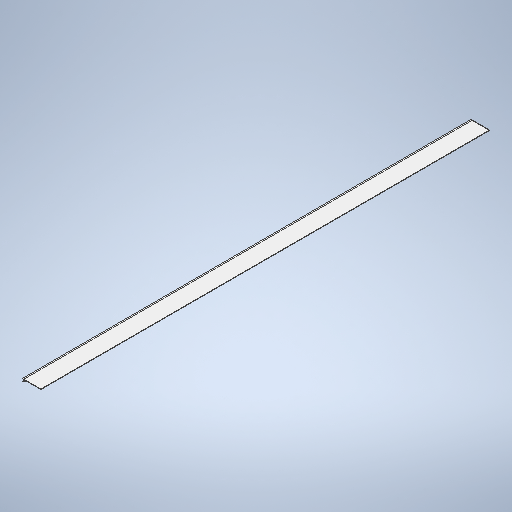
# Autodesk Inventor part: Drip_Edge_For_Side
Saved by Autodesk Inventor 2025 (Build 290162010, 162A)
## iProperties
Created: 2024-09-15
Part Number: Drip_Edge_For_Side
Material: Aluminum 6061
Document SubType Name: Modeling
Designer: Tom
Density: 2.7 g/cm^3
Appearance: White
Author: Tom
Autodesk Inventor part; units mm, degrees
ref_plane "YZ Plane" through (0, 0, 0) normal (1, 0, 0) x (0, 1, 0)
ref_plane "XZ Plane" through (0, 0, 0) normal (0, 1, 0) x (-1, 0, 0)
ref_plane "XY Plane" through (0, 0, 0) normal (0, 0, 1) x (1, 0, 0)
sketch "Sketch1" plane through (0, 0, 0) normal (0, 0, 1) x (1, 0, 0)
  line L0 (152.4, -3.175) -> (152.4, 0)
  line L1 (152.4, 0) -> (0, 0)
  line L2 (0, 0) -> (9.525, -8.4582)
  line L3 (9.525, -8.4582) -> (9.525, -16.9164)
  line L4 (9.525, -16.9164) -> (0, -22.655)
  line L5 (1.6385, -25.3746) -> (12.7, -18.7102)
  line L6 (12.7, -18.7102) -> (12.7, -7.0315)
  line L7 (12.7, -7.0315) -> (8.3571, -3.175)
  line L8 (8.3571, -3.175) -> (152.4, -3.175)
  line L9 (1.6385, -25.3746) -> (0, -22.655)
  line L10 (0, 0) -> (0, -22.655)
  dimension "d49" = 3.175
  dimension "d50" = 3.175
  dimension "d51" = 3.175
  dimension "d52" = 3.175
  dimension "d54" = 8.4582
  dimension "d55" = 8.4582
  dimension "d61" = 8.4582
  dimension "d62" = 152.4
  dimension "d64" = 12.7
  constraints: 22 end point, 4 parallel, 2 perpendicular, 1 coincident, 1 horizontal, 1 vertical
  measures "d49" distance between parallel lines of L1 L8
  measures "d50" distance between parallel lines of L3 L6
  measures "d51" distance between parallel lines of L2 L7
  measures "d52" distance between parallel lines of L4 L5
  measures "d54" distance of L3.end L2.end
  measures "d55" vertical distance of L5.start L3.end
  measures "d61" vertical distance of L2.end L1.end
  measures "d62" distance of L0.end L1.end
  measures "d64" distance from line of L6 L1.end
extrude "Extrusion2" add sketch "Sketch1" along normal blind 3709.1747 contours L8 L7 L6 L5 L9 L4 L3 L2 L1 L0
body "Solid2"
